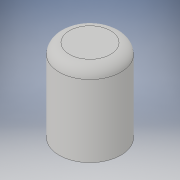
# Autodesk Inventor part: Button
Saved by Autodesk Inventor 2019.3 (Build 233278000, 278)
## iProperties
Created: 2019-03-10
Part Number: Button
Material: Generic
Document SubType Name: Modeling
Designer: Jared
Density: 1 g/cm^3
Appearance: Default
Author: Jared
Autodesk Inventor part; units mm, degrees
ref_plane "YZ Plane" through (0, 0, 0) normal (1, 0, 0) x (0, 1, 0)
ref_plane "XZ Plane" through (0, 0, 0) normal (0, 1, 0) x (-1, 0, 0)
ref_plane "XY Plane" through (0, 0, 0) normal (0, 0, 1) x (1, 0, 0)
sketch "Sketch1" plane through (0, 0, 0) normal (0, 1, 0) x (-1, 0, 0)
  circle A0 centre (0, 0) radius 3
  dimension "d0" = 6
  constraints: 1 centre point, 1 coincident
  measures "d0" diameter of A0
extrude "Extrusion1" add sketch "Sketch1" along normal blind 8
sketch "Sketch2" plane through (0, 0, 0) normal (0, -1, 0) x (1, 0, 0)
  line L0 (-1.375, -1.375) -> (1.375, -1.375)
  line L1 (1.375, -1.375) -> (1.375, 1.375)
  line L2 (1.375, 1.375) -> (-1.375, 1.375)
  line L3 (-1.375, 1.375) -> (-1.375, -1.375)
  line L4 (-1.375, -1.375) -> (1.375, 1.375) construction
  line L5 (1.375, -1.375) -> (-1.375, 1.375) construction
  point P0 (0, 0)
  dimension "d3" = 2.75
  dimension "d4" = 2.75
  constraints: 12 end point, 2 midpoint, 2 parallel, 1 horizontal, 1 perpendicular
  measures "d3" distance of L2.end L1.end
  measures "d4" distance of L1.end L0.end
extrude "Extrusion2" cut sketch "Sketch2" against normal blind 2.5
fillet "Fillet1" radius 1 1 edges at (3, 8, 0)
body "Solid1"
